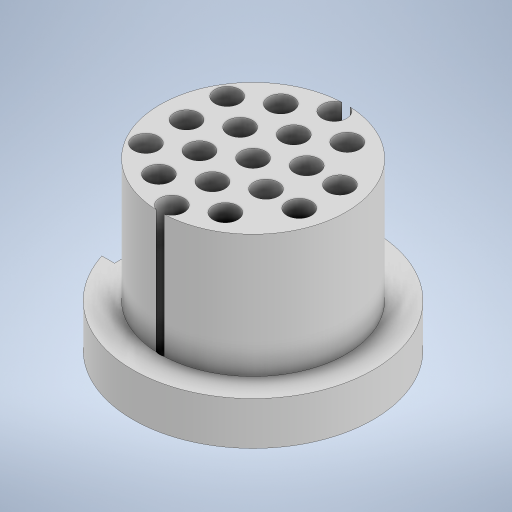
# Autodesk Inventor part: inner Part of Adaptor
Saved by Autodesk Inventor 2023 (Build 270158000, 158)
## iProperties
Created: 2022-10-16
Part Number: inner Part of Adaptor
Material: Generic
Document SubType Name: Modeling
Designer: rayle
Density: 1 g/cm^3
Appearance: Default
Author: rayle
Autodesk Inventor part; units mm, degrees
ref_plane "YZ Plane" through (0, 0, 0) normal (1, 0, 0) x (0, 1, 0)
ref_plane "XZ Plane" through (0, 0, 0) normal (0, 1, 0) x (-1, 0, 0)
ref_plane "XY Plane" through (0, 0, 0) normal (0, 0, 1) x (1, 0, 0)
sketch "Sketch1" plane through (0, 0, 0) normal (0, 1, 0) x (-1, 0, 0)
  point P0 (0, 0)
sketch "Sketch2" plane through (0, 0, 0) normal (0, 1, 0) x (-1, 0, 0)
  line L0 (0, -0.6) -> (0, -2.7)
  line L1 (0, -2.7) -> (0, -3.3)
  line L2 (0, -3.9) -> (0, -6)
  line L3 (0, -6) -> (0, -6.6)
  line L4 (0, 0.6) -> (0, 3.3)
  line L5 (0, 3.9) -> (0, 6.6)
  line L6 (0, -0.6) -> (0, -1.65)
  line L7 (0, -0.6) -> (0, -1.65)
  line L8 (0, -1.65) -> (2.7, -1.65)
  line L9 (2.7, -1.65) -> (2.7, -3.75)
  line L10 (2.7, -3.75) -> (2.7, -4.95)
  line L11 (2.7, -1.05) -> (2.7, 1.05)
  line L12 (2.7, 1.05) -> (2.7, 1.65)
  line L13 (2.7, 2.25) -> (2.7, 4.95)
  line L14 (2.7, 0) -> (5.4, 0)
  line L15 (5.4, 0) -> (5.4, -3.3)
  line L16 (5.4, 0) -> (5.4, 3.3)
  line L17 (0, -1.65) -> (-2.7, -1.65)
  line L18 (-2.7, -1.65) -> (-2.7, -4.35)
  line L19 (-2.7, -4.35) -> (-2.7, -4.95)
  line L20 (-2.7, -1.65) -> (-2.7, 1.65)
  line L21 (-2.7, 1.65) -> (-2.7, 4.95)
  line L22 (-2.7, -1.65) -> (-5.4, -1.65)
  line L23 (-2.7, 1.65) -> (-5.4, 1.65)
  circle A0 centre (0, -6.6) radius 1
  circle A1 centre (2.7, -4.95) radius 1
  circle A2 centre (-2.7, -4.95) radius 1
  circle A3 centre (0, -3.3) radius 1
  circle A4 centre (5.4, -3.3) radius 1
  circle A5 centre (2.7, -1.65) radius 1
  circle A6 centre (-2.7, -1.65) radius 1
  circle A7 centre (-5.4, -1.65) radius 1
  circle A8 centre (0, 0) radius 1
  circle A9 centre (5.4, 0) radius 1
  circle A10 centre (2.7, 1.65) radius 1
  circle A11 centre (5.4, 3.3) radius 1
  circle A12 centre (0, 3.3) radius 1
  circle A13 centre (-2.7, 1.65) radius 1
  circle A14 centre (-5.4, 1.65) radius 1
  circle A15 centre (-2.7, 4.95) radius 1
  circle A16 centre (2.7, 4.95) radius 1
  circle A17 centre (0, 6.6) radius 1
  circle A18 centre (0, 0) radius 9.75
  line L24 (9.75, 0) -> (8.25, 0)
  line L25 (8.25, 0) -> (8.25, 3)
  line L26 (8.25, 3) -> (10.1008, 3)
  line L27 (8.25, 0) -> (8.25, -3)
  line L28 (8.25, -3) -> (10.4334, -3)
  point P0 (-2, 10.0571)
  point P1 (2, 10.0571)
  point P2 (9.277, 3)
  point P3 (9.277, -3)
  dimension "d127" = 19.5
  dimension "d53" = 2.1
  dimension "d54" = 0.6
  dimension "d56" = 2.1
  dimension "d57" = 0.6
  dimension "d59" = 2.7
  dimension "d61" = 2.7
  dimension "d63" = 1.05
  dimension "d64" = 2.7
  dimension "d66" = 2.1
  dimension "d67" = 1.2
  dimension "d69" = 2.1
  dimension "d70" = 0.6
  dimension "d72" = 2.7
  dimension "d74" = 2.7
  dimension "d78" = 2.7
  dimension "d80" = 2.7
  dimension "d81" = 0.6
  dimension "d85" = 2.7
  dimension "d87" = 2.7
  dimension "d91" = 2
  dimension "d92" = 2
  dimension "d93" = 2
  dimension "d94" = 2
  dimension "d95" = 2
  dimension "d96" = 2
  dimension "d97" = 2
  dimension "d98" = 2
  dimension "d99" = 2
  dimension "d100" = 2
  dimension "d101" = 2
  dimension "d102" = 2
  dimension "d103" = 2
  dimension "d104" = 2
  dimension "d105" = 2
  dimension "d106" = 2
  dimension "d107" = 2
  dimension "d108" = 2
  dimension "d128" = 1.5
  dimension "d129" = 3
  dimension "d130" = 3
  constraints: 58 end point, 18 centre point, 15 vertical, 9 coincident, 6 perpendicular, 4 point on line, 2 horizontal, 2 midpoint, 1 collinear, 3 other
  measures "d53" distance of L0.start L0.end
  measures "d54" distance of L0.end L1.end
  measures "d56" distance of L2.start L2.end
  measures "d57" distance of L2.end L3.end
  measures "d59" distance of L4.start L4.end
  measures "d61" distance of L5.start L5.end
  measures "d63" distance of L0.start L17.start
  measures "d64" distance of L17.start L8.end
  measures "d66" distance of L9.start L10.start
  measures "d67" distance of L10.start L10.end
  measures "d69" distance of L11.start L11.end
  measures "d70" distance of L11.end L12.end
  measures "d72" distance of L13.start L13.end
  measures "d74" distance of L14.start L14.end
  measures "d78" distance of L17.start L17.end
  measures "d80" distance of L18.start L18.end
  measures "d81" distance of L18.end L19.end
  measures "d85" distance of L18.start L22.end
  measures "d87" distance of L23.start L23.end
  measures "d91" diameter of A0
  measures "d92" diameter of A1
  measures "d93" diameter of A2
  measures "d94" diameter of A3
  measures "d95" diameter of A4
  measures "d96" diameter of A5
  measures "d97" diameter of A6
  measures "d98" diameter of A7
  measures "d99" diameter of A8
  measures "d100" diameter of A9
  measures "d101" diameter of A10
  measures "d102" diameter of A11
  measures "d103" diameter of A12
  measures "d104" diameter of A13
  measures "d105" diameter of A14
  measures "d106" diameter of A15
  measures "d107" diameter of A16
  measures "d108" diameter of A17
  measures "d128" distance of L24.start L24.end
  measures "d129" distance of L24.end L25.end
  measures "d130" distance of L24.end L27.end
extrude "Extrusion1" add sketch "Sketch2" along normal blind 3.5 contours L26 L25 L27 L28 A18
sketch "Sketch3" plane through (0, 3.5, 0) normal (0, 1, 0) x (-1, 0, 0)
  circle A0 centre (0, 0) radius 7.55
  line L0 (0, -0.6) -> (0, -2.7)
  line L1 (0, -2.7) -> (0, -3.3)
  line L2 (0, -3.9) -> (0, -6)
  line L3 (0, -6) -> (0, -6.6)
  line L4 (0, 0.6) -> (0, 3.3)
  line L5 (0, 3.9) -> (0, 6.6)
  line L6 (0, -0.6) -> (0, -1.65)
  line L7 (0, -0.6) -> (0, -1.65)
  line L8 (0, -1.65) -> (2.7, -1.65)
  line L9 (2.7, -1.65) -> (2.7, -3.75)
  line L10 (2.7, -3.75) -> (2.7, -4.95)
  line L11 (2.7, -1.05) -> (2.7, 1.05)
  line L12 (2.7, 1.05) -> (2.7, 1.65)
  line L13 (2.7, 2.25) -> (2.7, 4.95)
  line L14 (2.7, 0) -> (5.4, 0)
  line L15 (5.4, 0) -> (5.4, -3.3)
  line L16 (5.4, 0) -> (5.4, 3.3)
  line L17 (0, -1.65) -> (-2.7, -1.65)
  line L18 (-2.7, -1.65) -> (-2.7, -4.35)
  line L19 (-2.7, -4.35) -> (-2.7, -4.95)
  line L20 (-2.7, -1.65) -> (-2.7, 1.65)
  line L21 (-2.7, 1.65) -> (-2.7, 4.95)
  line L22 (-2.7, -1.65) -> (-5.4, -1.65)
  line L23 (-2.7, 1.65) -> (-5.4, 1.65)
  circle A1 centre (0, -6.6) radius 1
  circle A2 centre (-2.7, -4.95) radius 1
  circle A3 centre (0, -3.3) radius 1
  circle A4 centre (2.7, -4.95) radius 1
  circle A5 centre (5.4, -3.3) radius 1
  circle A6 centre (2.7, -1.65) radius 1
  circle A7 centre (-2.7, -1.65) radius 1
  circle A8 centre (-5.4, -1.65) radius 1
  circle A9 centre (5.4, 0) radius 1
  circle A10 centre (0, 0) radius 1
  circle A11 centre (2.7, 1.65) radius 1
  circle A12 centre (-2.7, 1.65) radius 1
  circle A13 centre (-5.4, 1.65) radius 1
  circle A14 centre (0, 3.3) radius 1
  circle A15 centre (5.4, 3.3) radius 1
  circle A16 centre (2.7, 4.95) radius 1
  circle A17 centre (-2.7, 4.95) radius 1
  circle A18 centre (0, 6.6) radius 1
  point P0 (-0.3339, 7.5426)
  point P1 (-0.3339, -7.5426)
  point P2 (0.3339, -7.5426)
  point P3 (0.3339, 7.5426)
  dimension "d12" = 2.1
  dimension "d13" = 0.6
  dimension "d15" = 2.1
  dimension "d16" = 0.6
  dimension "d18" = 2.7
  dimension "d20" = 2.7
  dimension "d22" = 1.05
  dimension "d23" = 2.7
  dimension "d25" = 2.1
  dimension "d26" = 1.2
  dimension "d28" = 2.1
  dimension "d29" = 0.6
  dimension "d31" = 2.7
  dimension "d33" = 2.7
  dimension "d37" = 2.7
  dimension "d39" = 2.7
  dimension "d40" = 0.6
  dimension "d44" = 2.7
  dimension "d46" = 2.7
  dimension "d109" = 2
  dimension "d110" = 2
  dimension "d111" = 2
  dimension "d112" = 2
  dimension "d113" = 2
  dimension "d114" = 2
  dimension "d115" = 2
  dimension "d116" = 2
  dimension "d117" = 2
  dimension "d118" = 2
  dimension "d119" = 2
  dimension "d120" = 2
  dimension "d121" = 2
  dimension "d122" = 2
  dimension "d123" = 2
  dimension "d124" = 2
  dimension "d125" = 2
  dimension "d126" = 2
  constraints: 48 end point, 19 centre point, 14 vertical, 9 coincident, 4 point on line, 3 perpendicular, 2 midpoint, 1 collinear, 1 horizontal
  measures "d12" distance of L0.start L0.end
  measures "d13" distance of L0.end L1.end
  measures "d15" distance of L2.start L2.end
  measures "d16" distance of L2.end L3.end
  measures "d18" distance of L4.start L4.end
  measures "d20" distance of L5.start L5.end
  measures "d22" distance of L0.start L6.end
  measures "d23" distance of L6.end L8.end
  measures "d25" distance of L9.start L9.end
  measures "d26" distance of L9.end L10.end
  measures "d28" distance of L11.start L11.end
  measures "d29" distance of L11.end L12.end
  measures "d31" distance of L13.start L13.end
  measures "d33" distance of L14.start L14.end
  measures "d37" distance of L6.end L17.end
  measures "d39" distance of L18.start L18.end
  measures "d40" distance of L18.end L19.end
  measures "d44" distance of L18.start L22.end
  measures "d46" distance of L21.start L23.end
  measures "d109" diameter of A1
  measures "d110" diameter of A2
  measures "d111" diameter of A3
  measures "d112" diameter of A4
  measures "d113" diameter of A5
  measures "d114" diameter of A6
  measures "d115" diameter of A7
  measures "d116" diameter of A8
  measures "d117" diameter of A9
  measures "d118" diameter of A10
  measures "d119" diameter of A11
  measures "d120" diameter of A12
  measures "d121" diameter of A13
  measures "d122" diameter of A14
  measures "d123" diameter of A15
  measures "d124" diameter of A16
  measures "d125" diameter of A17
  measures "d126" diameter of A18
extrude "Extrusion2" add sketch "Sketch3" along normal blind 10 contours A0 A1 L2 A3 L0 A10 L4 A14 L5 A18 | A18 L5 A14 L4 A10 L0 A3 L2 A1 A0
body "Solid1"
